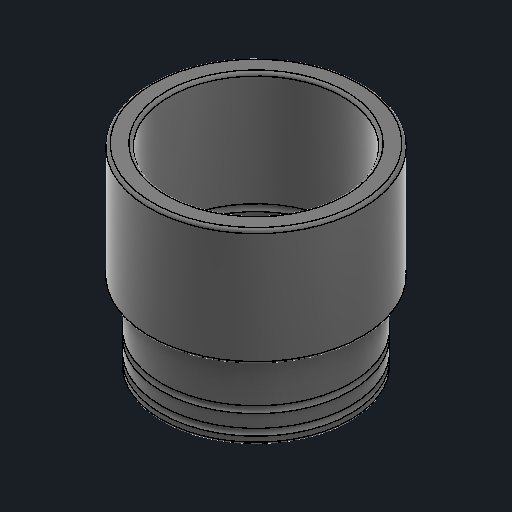
# Autodesk Inventor part: Tapered Vac Fitting
Saved by Autodesk Inventor 2026.2 (Build 302298000, 298)
## iProperties
Created: 2026-07-13
Part Number: Tapered Vac Fitting
Material: PVC, Unplasticized
Document SubType Name: Modeling
Designer: Joshua Eah
Density: 1.29 g/cm^3
Appearance: Smooth - Black
Author: Joshua Eah
Autodesk Inventor part; units mm, degrees
ref_plane "YZ Plane" through (0, 0, 0) normal (1, 0, 0) x (0, 1, 0)
ref_plane "XZ Plane" through (0, 0, 0) normal (0, 1, 0) x (-1, 0, 0)
ref_plane "XY Plane" through (0, 0, 0) normal (0, 0, 1) x (1, 0, 0)
sketch "Sketch4" plane through (0, 0, 0) normal (0, 0, 1) x (1, 0, 0)
  line L0 (0, 0) -> (0, 50)
  line L1 (0, 50) -> (27.225, 50)
  line L2 (24.225, 50) -> (24.225, 0)
  line L3 (24.225, 0) -> (0, 0)
  line L4 (22.25, 50) -> (22.25, 0)
  line L5 (20.25, 0) -> (20.25, 10)
  line L6 (20.25, 10) -> (22.25, 10)
  circle A0 centre (24.225, 3) radius 0.875
  circle A1 centre (22.25, 15) radius 0.875
  circle A2 centre (24.225, 8) radius 0.875
  line L7 (27.225, 50) -> (27.225, 20)
  line L8 (27.225, 20) -> (24.225, 20)
  circle A3 centre (22.25, 20) radius 0.875
  point P0 (24.225, 2.125)
  point P1 (24.225, 3.875)
  point P2 (22.25, 15.875)
  point P3 (22.25, 14.125)
  point P4 (24.225, 7.125)
  point P5 (24.225, 8.875)
  point P6 (22.25, 20.875)
  point P7 (22.25, 19.125)
  dimension "d56" = 48.45
  dimension "d57" = 44.5
  dimension "d59" = 10
  dimension "d60" = 2
  dimension "d61" = 1.75
  dimension "d63" = 5
  dimension "d69" = 5
  dimension "d74" = 3
  dimension "d75" = 40
  dimension "d76" = 30
  dimension "d77" = 3
  dimension "d80" = 5
  constraints: 18 end point, 8 point on line, 4 centre point, 4 perpendicular, 4 vertical, 1 coincident, 1 equal radius, 1 horizontal, 4 other
  measures "d56" diameter of L2 L0
  measures "d57" diameter of L4 L0
  measures "d59" distance of L5.start L5.end
  measures "d60" distance of L5.end L6.end
  measures "d61" diameter of A0
  measures "d63" distance from line of L6 A1.centre
  measures "d69" distance of A0.centre A2.centre
  measures "d74" distance from line of L3 A0.centre
  measures "d75" distance between parallel lines of L6 L1
  measures "d76" distance of L1.end L7.end
  measures "d77" distance of L7.end L8.end
  measures "d80" distance of A1.centre A3.centre
revolve "Revolution2" add sketch "Sketch4" angle 360 about axis through (0, 0, 0) along (0, 1, 0) contours L5 L6 L4 L3 | L1 L2 A2 A0 L3 L4 A1 A3 | L1 L7 L8 L2
fillet "Fillet4" radius 0.8 6 edges at (-22.25, 50, 0) (-24.225, 0, 0) (-20.25, 0, 0) (-27.225, 50, 0) (-27.225, 20, 0) (-24.225, 20, 0)
fillet "Fillet5" radius 0.4 2 edges at (-22.25, 10, 0) (-20.25, 10, 0)
body "Solid2"
